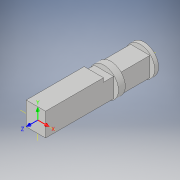
# Autodesk Inventor part: link_4
Saved by Autodesk Inventor 2019 (Build 230136000, 136)
## iProperties
Created: 2020-08-30
Part Number: link_4
Material: Generic
Document SubType Name: Modeling
Designer: Daniel
Density: 1 g/cm^3
Appearance: Default
Author: Daniel
Autodesk Inventor part; units mm, degrees
ref_plane "XZ Plane" through (0, 0, 0) normal (0, 1, 0) x (-1, 0, 0)
sketch "Sketch1" plane through (0, 0, 0) normal (0, 0, 1) x (1, 0, 0)
  line L0 (-20, -20) -> (20, -20)
  line L1 (20, -20) -> (20, 28)
  line L2 (20, 28) -> (-20, 28)
  line L3 (-20, 28) -> (-20, -20)
  line L4 (-20, -20) -> (20, 28) construction
  line L5 (20, -20) -> (-20, 28) construction
  line L6 (0, -29.6) -> (0, 37.6) projected
  point P0 (0, 0)
  point P1 (0, 4)
  dimension "d0" = 20
  dimension "d1" = 28
  dimension "d2" = 40
  constraints: 12 end point, 3 midpoint, 2 parallel, 1 horizontal, 1 perpendicular
  measures "d0" distance from line of L0 point (0, 0)
  measures "d1" distance from line of L2 point (0, 0)
  measures "d2" distance between parallel lines of L1 L3
extrude "Extrusion1" add sketch "Sketch1" along normal blind 4 and the other way blind 116
sketch "Sketch3" plane through (0, 0, -116) normal (0, 0, -1) x (-1, 0, 0)
  line L0 (-20, -20) -> (20, -20)
  line L1 (20, -20) -> (20, 20)
  line L2 (20, 20) -> (-20, 20)
  line L3 (-20, 20) -> (-20, -20)
  line L4 (-20, -20) -> (20, 20) construction
  line L5 (20, -20) -> (-20, 20) construction
  line L6 (0, -29.6) -> (0, 37.6) projected
  line L7 (-20, -20) -> (20, -20) projected
  line L8 (20, -20) -> (20, 28) projected
  line L9 (20, 28) -> (-20, 28) projected
  point P0 (0, 0)
  point P1 (0, 0)
  point P2 (0, 0)
  dimension "d16" = 8
  constraints: 12 end point, 3 midpoint, 2 collinear, 2 parallel, 1 horizontal, 1 perpendicular, 1 point on line
  measures "d16" distance between parallel lines of L9 L2
extrude "Extrusion3" add sketch "Sketch3" along normal blind 96 contours L3 L2 L6 L0 | L6 L2 L1 L0
ref_plane "Work Plane1" through (0, 0, -144) normal (0, 0, 1) x (1, 0, 0)
sketch "Sketch4" plane through (0, 0, -144) normal (0, 0, 1) x (1, 0, 0)
  circle A0 centre (0, 0) radius 30
  dimension "d20" = 60
  constraints: 1 centre point, 1 coincident
  measures "d20" diameter of A0
extrude "Extrusion4" add sketch "Sketch4" along normal mid plane 14
sketch "Sketch5" plane through (0, 0, -212) normal (0, 0, -1) x (-1, 0, 0)
  circle A0 centre (0, 0) radius 30
  dimension "d23" = 60
  constraints: 1 centre point, 1 coincident
  measures "d23" diameter of A0
extrude "Extrusion5" add sketch "Sketch5" along normal blind 8
ref_plane "UCS4: YZ Plane" through (0, 0, 0) normal (1, 0, 0) x (0, 1, 0)
ref_plane "UCS4: XZ Plane" through (0, 0, 0) normal (0, 1, 0) x (0, 0, 1)
ref_plane "UCS4: XY Plane" through (0, 0, 0) normal (0, 0, 1) x (1, 0, 0)
body "Solid1"
